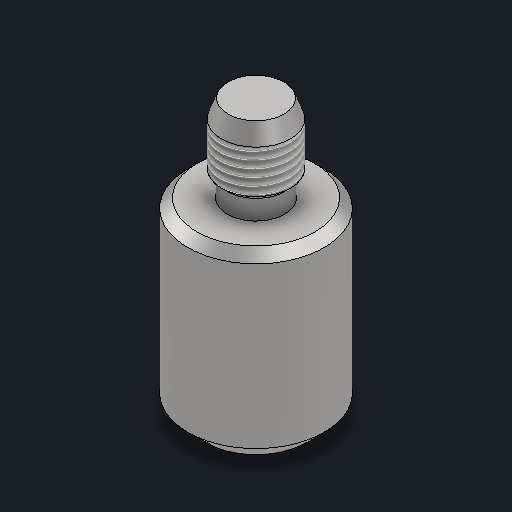
# Autodesk Inventor part: 0.375 Shaft
Saved by Autodesk Inventor 2025.1 (Build 291241020, 241B)
## iProperties
Created: 2025-05-15
Part Number: 0.375 Shaft
Material: Stainless Steel
Document SubType Name: Modeling
Designer: Joshua Eah
Density: 8 g/cm^3
Appearance: Semi-Polished
Author: Joshua Eah
Autodesk Inventor part; units mm, degrees
ref_plane "YZ Plane" through (0, 0, 0) normal (1, 0, 0) x (0, 1, 0)
ref_plane "XZ Plane" through (0, 0, 0) normal (0, 1, 0) x (-1, 0, 0)
ref_plane "XY Plane" through (0, 0, 0) normal (0, 0, 1) x (1, 0, 0)
sketch "Sketch1" plane through (0, 0, 0) normal (0, 1, 0) x (-1, 0, 0)
  circle A0 centre (0, 0) radius 4.7625
  line L0 (0.635, 4.7625) -> (-0.635, 4.7625)
  line L1 (-0.635, 4.7625) -> (-0.635, -4.7625)
  line L2 (-0.635, -4.7625) -> (0.635, -4.7625)
  line L3 (0.635, -4.7625) -> (0.635, 4.7625)
  line L4 (0.635, 4.7625) -> (-0.635, -4.7625) construction
  line L5 (-0.635, 4.7625) -> (0.635, -4.7625) construction
  point P0 (0.635, -4.72)
  point P1 (0.635, 4.72)
  point P2 (-0.635, 4.72)
  point P3 (-0.635, -4.72)
  dimension "d0" = 9.525
  dimension "d9" = 1.27
  constraints: 12 end point, 2 midpoint, 2 parallel, 1 centre point, 1 coincident, 1 horizontal, 1 perpendicular, 1 tangent
  measures "d0" diameter of A0
  measures "d9" distance of L2.end L1.end
extrude "Extrusion1" add sketch "Sketch1" along normal blind 13.081 contours A0 L3 | L3 A0 L1 | L1 A0
sketch "Sketch2" plane through (0, 13.081, 0) normal (0, 1, 0) x (1, 0, 0)
  circle A0 centre (0, 0) radius 2.0003
  dimension "d3" = 4.0005
  constraints: 1 centre point, 1 coincident
  measures "d3" diameter of A0
extrude "Extrusion2" add sketch "Sketch2" along normal blind 1.778
sketch "Sketch3" plane through (0, 14.859, 0) normal (0, 1, 0) x (1, 0, 0)
  circle A0 centre (0, 0) radius 2.413
  dimension "d19" = 4.826
  constraints: 1 centre point, 1 coincident
  measures "d19" diameter of A0
extrude "Extrusion4" add sketch "Sketch3" along normal blind 4.2545
extrude "Extrusion3" cut sketch "Sketch1" along normal blind 1.27 contours L3 A0 L1
chamfer "Chamfer2" distance 0.635 angle 45 1 edges at (4.7625, 13.081, 0)
chamfer "Chamfer1" distance 1.27 angle 45 3 edges at (-3.5851, 0, -3.1351) (-3.5851, 0, 3.1351) (4.7625, 0, 0)
chamfer "Chamfer3" distance 0.4064 angle 45 1 edges at (-2.0003, 14.859, 0)
chamfer "Chamfer4" distance 1.27 angle 20 1 edges at (-2.413, 19.1135, 0) measured on face at (2.4052, 17.6953, 0.1942)
thread "Thread3" size "10-48 UNS" class "2A" standard "ANSI Unified Screw Threads" length 6.0325
body "Solid1"
